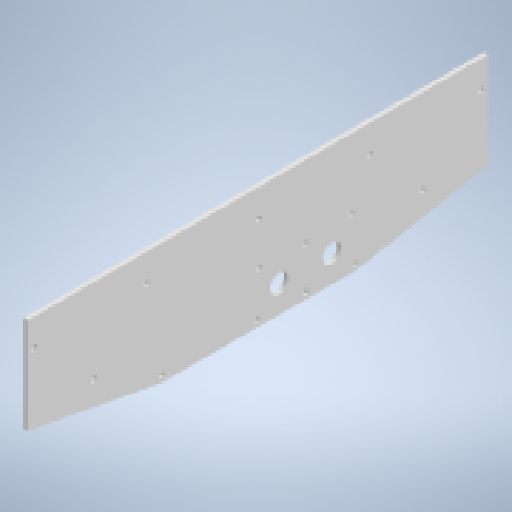
# Autodesk Inventor part: Outside Chassi Plate low 2.0
Saved by Autodesk Inventor 2023 (Build 270158000, 158)
## iProperties
Created: 2022-09-05
Part Number: Outside Chassi Plate low 2.0
Material: Generic
Document SubType Name: Modeling
Designer: deli
Density: 1 g/cm^3
Appearance: Default
Author: deli
Autodesk Inventor part; units mm, degrees
ref_plane "YZ Plane" through (0, 0, 0) normal (1, 0, 0) x (0, 1, 0)
ref_plane "XZ Plane" through (0, 0, 0) normal (0, 1, 0) x (-1, 0, 0)
ref_plane "XY Plane" through (0, 0, 0) normal (0, 0, 1) x (1, 0, 0)
sketch "Sketch1" plane through (0, 0, 0) normal (1, 0, 0) x (0, 1, 0)
  line L0 (-213.0456, 506.9498) -> (-285.8918, 506.9498)
  line L1 (-285.8918, 506.9498) -> (-304.9582, 406.3261)
  line L2 (-213.0456, 156.9498) -> (-285.8918, 156.9498)
  circle A0 centre (-277.0456, 456.9498) radius 2
  circle A1 centre (-277.0456, 456.9498) radius 48 construction
  arc A2 (-265.1215, 456.4048) -> (-288.9629, 457.629) centre (-277.0456, 456.9498) ccw construction
  circle A3 centre (-277.0456, 206.9498) radius 48 construction
  arc A4 (-288.901, 205.5596) -> (-265.1614, 208.0664) centre (-277.0456, 206.9498) ccw construction
  circle A5 centre (-277.0456, 206.9498) radius 2
  circle A6 centre (-284.2956, 315.7447) radius 7
  circle A7 centre (-284.2956, 275.607) radius 7
  circle A8 centre (-284.2956, 315.7447) radius 18.75 construction
  circle A9 centre (-284.2956, 275.607) radius 18.75 construction
  arc A10 (-297.0074, 316.4692) -> (-271.5765, 315.1634) centre (-284.2956, 315.7447) ccw construction
  arc A11 (-271.6191, 276.7981) -> (-296.9414, 274.1241) centre (-284.2956, 275.607) ccw construction
  line L3 (-265.1215, 456.4048) -> (-271.5765, 315.1634) construction
  line L4 (-297.0074, 316.4692) -> (-288.9629, 457.629) construction
  line L5 (-271.6191, 276.7981) -> (-265.1614, 208.0664) construction
  line L6 (-288.901, 205.5596) -> (-296.9414, 274.1241) construction
  circle A12 centre (-268.1617, 295.6759) radius 2
  circle A13 centre (-300.4296, 295.6759) radius 2
  circle A14 centre (-300.0456, 332.8474) radius 2
  circle A15 centre (-300.0456, 258.5044) radius 2
  circle A16 centre (-266.1266, 261.1002) radius 2
  circle A17 centre (-234.0456, 501.9498) radius 2
  circle A18 centre (-234.0456, 161.9498) radius 2
  arc A19 (-305.0456, 229.9036) -> (-305.0456, 229.9036) centre (-282.2956, 229.9036) ccw
  line L7 (-305.0456, 258.5044) -> (-305.0456, 229.9036)
  arc A20 (-304.9582, 406.3261) -> (-305.0456, 405.3952) centre (-300.0456, 405.3952) ccw
  line L8 (-305.0456, 405.3952) -> (-305.0456, 229.9036)
  line L9 (-285.8918, 156.9498) -> (-304.9582, 257.5735)
  circle A21 centre (-266.8437, 331.1068) radius 2
  arc A22 (-305.0456, 258.5044) -> (-304.9582, 257.5735) centre (-300.0456, 258.5044) ccw
  circle A23 centre (-234.0456, 246.9498) radius 2
  line L10 (-213.0456, 506.9498) -> (-213.0456, 156.9498)
  line L11 (-213.0456, 193.3998) -> (-213.0456, 156.9498)
  circle A24 centre (-234.0456, 416.9498) radius 2
  circle A25 centre (-234.0456, 331.9498) radius 2
  circle A26 centre (-300.0456, 405.3952) radius 2
  point P0 (0, 0)
  dimension "d43" = 350
  dimension "d44" = 4
  dimension "d46" = 96
  dimension "d47" = 23.8732
  dimension "d48" = 96
  dimension "d49" = 4
  dimension "d51" = 23.8732
  dimension "d54" = 50
  dimension "d55" = 50
  dimension "d58" = 14
  dimension "d59" = 14
  dimension "d60" = 37.5
  dimension "d61" = 37.5
  dimension "d62" = 25.4648
  dimension "d63" = 25.4648
  dimension "d64" = 179.355
  dimension "d65" = 179.355
  dimension "d66" = 178.679
  dimension "d67" = 178.679
  dimension "d68" = 141.3888
  dimension "d70" = 69.0344
  dimension "d74" = 4
  dimension "d75" = 4
  dimension "d77" = 4
  dimension "d78" = 4
  dimension "d94" = 2.5
  dimension "d95" = 2.5
  dimension "d97" = 2.5
  dimension "d103" = 4
  dimension "d106" = 4
  dimension "d108" = 5
  dimension "d112" = 5
  dimension "d120" = 4
  dimension "d124" = 28
  dimension "d125" = 20.75
  dimension "d127" = 20.75
  dimension "d142" = 4
  dimension "d143" = 2.5
  dimension "d144" = 4
  dimension "d145" = 4
  dimension "d146" = 18
  dimension "d147" = 18
  dimension "d148" = 5
  dimension "d149" = 5
  dimension "d150" = 340
  dimension "d153" = 4
  dimension "d166" = 5
  dimension "d174" = 5
  dimension "d175" = 5
  dimension "d218" = 0
  dimension "d235" = 21
  dimension "d237" = 21
  dimension "d238" = 21
  dimension "d244" = 16
  dimension "d246" = 72.8462
  dimension "d247" = 72.8462
  dimension "d258" = 5
  dimension "d259" = 5
  dimension "d260" = 4
  dimension "d261" = 4
  dimension "d262" = 4
  dimension "d264" = 5
  dimension "d266" = 21
  dimension "d267" = 21
  constraints: 27 centre point, 24 end point, 15 point on circle, 14 tangent, 6 coincident, 6 vertical, 4 perpendicular, 3 concentric, 1 horizontal
  measures "d43" distance of L2.start L0.start
  measures "d44" diameter of A0
  measures "d46" diameter of A1
  measures "d47" diameter of A2
  measures "d48" diameter of A3
  measures "d49" diameter of A5
  measures "d51" diameter of A4
  measures "d54" distance from line of A0.centre L0
  measures "d55" distance from line of L2 A5.centre
  measures "d58" diameter of A6
  measures "d59" diameter of A7
  measures "d60" diameter of A8
  measures "d61" diameter of A9
  measures "d62" diameter of A10
  measures "d63" diameter of A11
  measures "d68" distance of L3.start L3.end
  measures "d70" distance of L5.start L5.end
  measures "d74" diameter of A14
  measures "d75" diameter of A13
  measures "d77" diameter of A12
  measures "d78" diameter of A16
  measures "d103" diameter of A17
  measures "d106" diameter of A18
  measures "d108" distance from line of L0 A17.centre
  measures "d112" distance from line of L2 A18.centre
  measures "d120" diameter of A15
  measures "d124" distance from line of A0.centre L7
  measures "d125" distance from line of L7 A6.centre
  measures "d127" distance from line of L7 A7.centre
  measures "d142" distance from line of L5 A16.centre
  measures "d144" distance from line of L3 A21.centre
  measures "d145" diameter of A21
  measures "d146" distance from line of A0.centre L1
  measures "d147" distance from line of L9 A3.centre
  measures "d148" radius of A20
  measures "d149" radius of A22
  measures "d150" distance of A18.centre A17.centre
  measures "d153" diameter of A23
  measures "d166" distance from line of L8 A14.centre
  measures "d218" horizontal distance of A0.centre A5.centre
  measures "d235" distance from line of L10 A17.centre
  measures "d237" distance from line of L11 A23.centre
  measures "d238" distance from line of L11 A18.centre
  measures "d244" distance edge to line of A1 L10
  measures "d246" distance of L2.start L2.end
  measures "d247" distance of L0.start L0.end
  measures "d260" diameter of A24
  measures "d261" diameter of A25
  measures "d262" diameter of A26
  measures "d264" distance from line of L8 A26.centre
  measures "d266" distance from line of L10 A24.centre
  measures "d267" distance from line of L10 A25.centre
extrude "Extrusion1" add sketch "Sketch1" along normal blind 3.175 contours L10 L2 L9 A19 A5 A22 L8 A20 L1 L0 | L9 A19 A5
body "Solid1"
